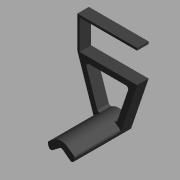
# Autodesk Inventor part: Part1
Saved by Autodesk Inventor 2019.3 (Build 233278000, 278)
## iProperties
Part Number: Part1
Material: Generic
Document SubType Name: Modeling
Designer: Frienddo
Appearance: Default
Author: Frienddo
Autodesk Inventor part; units mm, degrees
ref_plane "YZ Plane" through (0, 0, 0) normal (1, 0, 0) x (0, 1, 0)
ref_plane "XZ Plane" through (0, 0, 0) normal (0, 1, 0) x (-1, 0, 0)
ref_plane "XY Plane" through (0, 0, 0) normal (0, 0, 1) x (1, 0, 0)
sketch "Sketch1" plane through (0, 0, 0) normal (0, 0, 1) x (1, 0, 0)
  line L0 (52, 0) -> (0, 0)
  line L1 (0, 0) -> (0, -28)
  line L2 (52, -28) -> (2, -28)
  line L3 (2, -28) -> (2, -2)
  line L4 (2, -2) -> (52, -2)
  line L5 (52, -2) -> (52, 0)
  line L6 (0, -28) -> (16, -75.5)
  line L7 (16, -75.5) -> (26, -68)
  line L8 (26, -68) -> (36, -75.5)
  line L9 (36, -75.5) -> (52, -28)
  line L10 (26, -68) -> (26, -56.7382) construction
  dimension "d1" = 50
  dimension "d2" = 2
  dimension "d3" = 2
  dimension "d4" = 26
  dimension "d6" = 40
  dimension "d7" = 20
  dimension "d8" = 7.5
  constraints: 22 end point, 4 perpendicular, 2 equal length, 1 horizontal, 1 point on line, 1 symmetric about line, 1 vertical, 1 vertical alignment
  measures "d1" distance of L3.end L4.end
  measures "d2" distance between parallel lines of L1 L3
  measures "d3" distance between parallel lines of L0 L4
  measures "d4" distance between parallel lines of L4 L2
  measures "d6" distance from line of L2 L7.end
  measures "d7" distance of L8.end L6.end
  measures "d8" vertical distance of L7.end L8.end
extrude "Extrusion1" add sketch "Sketch1" along normal blind 10
sketch "Sketch2" plane through (0, 0, 10) normal (0, 0, 1) x (1, 0, 0)
  line L0 (16, -75.5) -> (26, -68) projected
  line L1 (26, -68) -> (36, -75.5) projected
  line L2 (26, -60.5) -> (38.0168, -69.5126)
  line L3 (52, -28) -> (36, -75.5) projected
  line L4 (36, -75.5) -> (38.0168, -69.5126)
  line L5 (26, -60.5) -> (13.9832, -69.5126)
  line L6 (0, -28) -> (16, -75.5) projected
  point P0 (0, 0)
  dimension "d13" = 6
  constraints: 6 end point, 2 parallel, 2 point on line, 1 collinear, 1 vertical alignment
  measures "d13" distance between parallel lines of L1 L2
extrude "Extrusion2" add sketch "Sketch2" along normal blind 40
sketch "Sketch3" plane through (0, 0, 10) normal (0, 0, 1) x (1, 0, 0)
  line L0 (26, -60.5) -> (38.0168, -69.5126) projected
  line L1 (38.0168, -69.5126) -> (52, -28) projected
  line L2 (52, -28) -> (2, -28) projected
  line L3 (2, -28) -> (2, -2) projected
  line L4 (2, -2) -> (52, -2) projected
  line L5 (52, -2) -> (52, 0) projected
  line L6 (52, 0) -> (0, 0) projected
  line L7 (0, 0) -> (0, -28) projected
  line L8 (0, -28) -> (13.9832, -69.5126) projected
  line L9 (13.9832, -69.5126) -> (26, -60.5) projected
  line L10 (6.9602, -33) -> (45.0398, -33)
  line L11 (45.0398, -33) -> (33.8048, -66.3536)
  line L12 (33.8048, -66.3536) -> (26, -60.5)
  line L13 (26, -60.5) -> (18.1952, -66.3536)
  line L14 (18.1952, -66.3536) -> (6.9602, -33)
  line L15 (52, -28) -> (2, -28) projected
  line L16 (38.0168, -69.5126) -> (52, -28) projected
  line L17 (0, -28) -> (13.9832, -69.5126) projected
  dimension "d14" = 5
  dimension "d15" = 5
  dimension "d16" = 5
  dimension "d17" = 0
  dimension "d18" = 0
  constraints: 10 end point, 3 parallel, 1 coincident, 1 horizontal
  measures "d14" distance between parallel lines of L16 L11
  measures "d15" distance between parallel lines of L2 L10
  measures "d16" distance between parallel lines of L8 L14
  measures "d17" distance between parallel lines of L9 L13
  measures "d18" distance between parallel lines of L0 L12
extrude "Extrusion3" cut sketch "Sketch3" against normal blind 40 contours L9 L14 L10 L11 L0
fillet "Fillet1" radius 10 2 edges at (0, -28, 5) (26, -60.5, 25)
fillet "Fillet2" radius 2 9 edges at (13.9832, -69.5126, 30) (16, -75.5, 25) (36, -75.5, 25) (26, -68, 25) (45.0398, -33, 5) (6.9602, -33, 5) (33.8048, -66.3536, 5) (18.1952, -66.3536, 5) (38.0168, -69.5126, 30)
body "Solid1"
